Autodesk Fusion 360 part; units mm, degrees
(part 2 of 2)
sketch "Sketch11 (2)" plane through (0, 0, 48.175) normal (0, 0, 1) x (-1, 0, 0)
  line L0 (-289.1, 4) -> (-319.1, 4)
  line L1 (-319.1, 4) -> (-319.1, 214)
  line L2 (-319.1, 214) -> (-289.1, 214)
  line L3 (-289.1, 214) -> (-289.1, 4)
  line L4 (-362.3136, 6.0325) -> (-387.8522, 6.0325)
  line L5 (-387.8522, 6.0325) -> (-387.8522, 6.8243)
  line L6 (-387.8522, 6.8243) -> (-400.7794, 11.0064)
  line L7 (-400.7794, 11.0064) -> (-404.4624, 13.6097)
  line L8 (-404.4624, 13.6097) -> (-401.1196, 16.5087)
  line L9 (-401.1196, 16.5087) -> (-390.396, 19.9107)
  arc A0 (-390.396, 19.9107) -> (-390.6158, 20.6037) centre (-390.5059, 20.2572) ccw
  line L10 (-390.6158, 20.6037) -> (-390.6158, 41.3132)
  line L11 (-390.6158, 41.3132) -> (-389.869, 42.5841)
  line L12 (-389.869, 42.5841) -> (-389.869, 50.7734)
  line L13 (-389.869, 50.7734) -> (-390.2857, 50.7734)
  spline S0 degree 5 poles (-390.2857, 50.7734) (-390.2828, 50.705) (-390.2784, 50.5702) (-390.2765, 50.3743) (-390.2832, 50.1256) (-390.3073, 49.8363) (-390.3474, 49.5695) (-390.4037, 49.326) (-390.4762, 49.1069) (-390.5636, 48.9124) (-390.6642, 48.7426) (-390.7753, 48.5968) (-390.8943, 48.4742) (-391.0189, 48.374) (-391.1473, 48.2953) (-391.2783, 48.2369) (-391.3847, 48.2058) (-391.4654, 48.1911) (-391.5195, 48.185) (-391.5467, 48.1829) knots -1 -1 -1 -1 -1 -1 -0.933333 -0.866667 -0.8 -0.733333 -0.666667 -0.6 -0.533333 -0.466667 -0.4 -0.333333 -0.266667 -0.2 -0.133333 -0.066667 0 0 0 0 0 0
  line L14 (-391.5467, 48.1829) -> (-396.3987, 48.1829)
  spline S1 degree 5 poles (-396.3987, 48.1829) (-396.4412, 48.1832) (-396.5253, 48.1877) (-396.6489, 48.2065) (-396.8084, 48.2552) (-396.9988, 48.3556) (-397.1797, 48.4948) (-397.3504, 48.6711) (-397.5092, 48.8811) (-397.6541, 49.1201) (-397.7831, 49.3821) (-397.8939, 49.6613) (-397.9848, 49.952) (-398.0548, 50.2496) (-398.104, 50.551) (-398.1331, 50.8546) (-398.1438, 51.1591) (-398.1381, 51.4639) (-398.1183, 51.7675) (-398.0869, 52.0681) (-398.0463, 52.3623) (-397.9988, 52.6463) (-397.946, 52.916) (-397.8892, 53.168) (-397.8286, 53.3999) (-397.7634, 53.611) (-397.6921, 53.8022) (-397.6123, 53.9753) (-397.5222, 54.1324) (-397.4199, 54.2753) (-397.3046, 54.4051) (-397.2016, 54.4991) (-397.1182, 54.5641) (-397.06, 54.605) (-397.0302, 54.6249) knots -1 -1 -1 -1 -1 -1 -0.966667 -0.933333 -0.9 -0.866667 -0.833333 -0.8 -0.766667 -0.733333 -0.7 -0.666667 -0.633333 -0.6 -0.566667 -0.533333 -0.5 -0.466667 -0.433333 -0.4 -0.366667 -0.333333 -0.3 -0.266667 -0.233333 -0.2 -0.166667 -0.133333 -0.1 -0.066667 -0.033333 0 0 0 0 0 0
  line L15 (-397.0302, 54.6249) -> (-391.0395, 54.6249)
  spline S2 degree 5 poles (-391.0395, 54.6249) (-391.0196, 54.5925) (-390.9803, 54.5265) (-390.9226, 54.4242) (-390.8482, 54.2808) (-390.7599, 54.0891) (-390.6766, 53.8841) (-390.5987, 53.6646) (-390.5263, 53.4305) (-390.4591, 53.1824) (-390.3967, 52.9217) (-390.3502, 52.7038) (-390.3173, 52.5354) (-390.2961, 52.4211) (-390.2857, 52.3633) knots -1 -1 -1 -1 -1 -1 -0.9 -0.8 -0.7 -0.6 -0.5 -0.4 -0.3 -0.2 -0.1 0 0 0 0 0 0
  line L16 (-390.2857, 52.3633) -> (-389.9496, 52.3633)
  line L17 (-389.9496, 52.3633) -> (-389.9505, 52.7079)
  line L18 (-389.9505, 52.7079) -> (-389.9505, 61.1725)
  spline S3 degree 5 poles (-389.9505, 61.1725) (-389.9574, 61.1784) (-389.9798, 61.1969) (-390.0205, 61.2265) (-390.0836, 61.2661) (-390.1737, 61.3196) (-390.2816, 61.3926) (-390.3919, 61.4876) (-390.5004, 61.6101) (-390.6038, 61.7602) (-390.6996, 61.933) (-390.7861, 62.1204) (-390.8622, 62.3125) (-390.927, 62.4996) (-390.9803, 62.6732) (-391.0219, 62.828) (-391.0519, 62.9611) (-391.0668, 63.0492) (-391.0729, 63.1049) (-391.0747, 63.1374) (-391.075, 63.1525) knots -0.77292 -0.77292 -0.77292 -0.77292 -0.77292 -0.77292 -0.75 -0.7 -0.65 -0.6 -0.55 -0.5 -0.45 -0.4 -0.35 -0.3 -0.25 -0.2 -0.15 -0.1 -0.05 0 0 0 0 0 0
  spline S4 degree 5 poles (-391.075, 63.1525) (-391.076, 63.2134) (-391.0784, 63.3525) (-391.0827, 63.5721) (-391.0896, 63.8767) (-391.1002, 64.2749) (-391.1133, 64.7103) (-391.1281, 65.1725) (-391.1444, 65.6712) (-391.1621, 66.2157) (-391.1809, 66.8139) (-391.2007, 67.4704) (-391.2214, 68.1843) (-391.243, 68.9483) (-391.2656, 69.7464) (-391.2898, 70.5518) (-391.3158, 71.3289) (-391.344, 72.0401) (-391.3744, 72.6507) (-391.4063, 73.1351) (-391.4381, 73.482) (-391.4674, 73.701) (-391.4903, 73.827) (-391.5015, 73.9279) (-391.4957, 74.0802) (-391.4698, 74.337) (-391.4238, 74.7122) (-391.3598, 75.1937) (-391.2811, 75.7505) (-391.1914, 76.3431) (-391.0939, 76.9317) (-390.9902, 77.4855) (-390.8799, 77.9908) (-390.7613, 78.4459) (-390.6319, 78.8575) (-390.4889, 79.2371) (-390.3301, 79.5967) (-390.1543, 79.9453) (-389.9622, 80.2849) (-389.7556, 80.6117) (-389.5364, 80.9182) (-389.306, 81.1959) (-389.0641, 81.4368) (-388.8079, 81.6362) (-388.5328, 81.7926) (-388.2336, 81.9077) (-387.9064, 81.9855) (-387.5495, 82.0319) (-387.165, 82.0543) (-386.7578, 82.0608) (-386.3345, 82.0591) (-385.9022, 82.0552) (-385.4676, 82.0533) (-385.0359, 82.0538) (-384.6109, 82.0543) (-384.1971, 82.0514) (-383.8005, 82.0428) (-383.4312, 82.0288) (-383.1037, 82.0144) (-382.8401, 82.0111) (-382.6594, 82.0319) (-382.5684, 82.0854) (-382.5488, 82.169) (-382.559, 82.2687) (-382.5646, 82.3519) (-382.563, 82.4147) (-382.5593, 82.4568) (-382.5568, 82.4778) knots -0.96593682 -0.96593682 -0.96593682 -0.96593682 -0.96593682 -0.96593682 -0.95384615 -0.93846154 -0.92307692 -0.90769231 -0.89230769 -0.87692308 -0.86153846 -0.84615385 -0.83076923 -0.81538462 -0.8 -0.78461538 -0.76923077 -0.75384615 -0.73846154 -0.72307692 -0.70769231 -0.69230769 -0.67692308 -0.66153846 -0.64615385 -0.63076923 -0.61538462 -0.6 -0.58461538 -0.56923077 -0.55384615 -0.53846154 -0.52307692 -0.50769231 -0.49230769 -0.47692308 -0.46153846 -0.44615385 -0.43076923 -0.41538462 -0.4 -0.38461538 -0.36923077 -0.35384615 -0.33846154 -0.32307692 -0.30769231 -0.29230769 -0.27692308 -0.26153846 -0.24615385 -0.23076923 -0.21538462 -0.2 -0.18461538 -0.16923077 -0.15384615 -0.13846154 -0.12307692 -0.10769231 -0.09230769 -0.07692308 -0.06153846 -0.04615385 -0.03076923 -0.01538462 0 0 0 0 0 0
  line L19 (-382.5568, 82.4778) -> (-382.673, 241.7066)
  line L20 (-382.673, 241.7066) -> (-366.4147, 241.7185)
  line L21 (-366.4147, 241.7185) -> (-366.3062, 93.0229)
  spline S5 degree 5 poles (-366.3062, 93.0229) (-366.2846, 93.0312) (-366.2188, 93.0608) (-366.0959, 93.134) (-365.8932, 93.2873) (-365.5824, 93.5536) (-365.1849, 93.8948) (-364.7435, 94.2418) (-364.2682, 94.5576) (-363.7673, 94.8157) (-363.2471, 95.0039) (-362.712, 95.1199) (-362.1658, 95.1683) (-361.6114, 95.1576) (-361.0522, 95.0971) (-360.4919, 94.9934) (-359.9353, 94.848) (-359.3882, 94.6593) (-358.8567, 94.4239) (-358.3475, 94.1384) (-357.8674, 93.8004) (-357.4229, 93.4106) (-357.0208, 92.9738) (-356.6667, 92.4989) (-356.3653, 91.9969) (-356.1199, 91.4799) (-355.9313, 90.9599) (-355.798, 90.4477) (-355.7154, 89.9513) (-355.6759, 89.4755) (-355.6713, 89.0222) (-355.6936, 88.5902) (-355.7373, 88.1762) (-355.8004, 87.7738) (-355.8859, 87.3747) (-355.9991, 86.9709) (-356.1458, 86.5564) (-356.3303, 86.1297) (-356.553, 85.6961) (-356.8092, 85.2687) (-357.091, 84.8639) (-357.389, 84.4988) (-357.6939, 84.1868) (-357.9979, 83.9346) (-358.2969, 83.7381) (-358.5478, 83.6074) (-358.7368, 83.5228) (-358.8668, 83.4687) (-358.9397, 83.4393) (-358.9561, 83.4328) knots -0.950494 -0.950494 -0.950494 -0.950494 -0.950494 -0.950494 -0.94 -0.92 -0.9 -0.88 -0.86 -0.84 -0.82 -0.8 -0.78 -0.76 -0.74 -0.72 -0.7 -0.68 -0.66 -0.64 -0.62 -0.6 -0.58 -0.56 -0.54 -0.52 -0.5 -0.48 -0.46 -0.44 -0.42 -0.4 -0.38 -0.36 -0.34 -0.32 -0.3 -0.28 -0.26 -0.24 -0.22 -0.2 -0.18 -0.16 -0.14 -0.12 -0.1 -0.08 -0.074178 -0.074178 -0.074178 -0.074178 -0.074178 -0.074178
  line L22 (-358.9561, 83.4328) -> (-359.4097, 83.2583)
  spline S6 degree 5 poles (-359.4097, 83.2583) (-359.4139, 83.2568) (-359.4729, 83.2345) (-359.5862, 83.1916) (-359.6985, 83.1487) (-359.81, 83.1056) (-359.9166, 83.0639) (-359.9697, 83.043) knots -0.041525 -0.041525 -0.041525 -0.041525 -0.041525 -0.041525 -0.04 -0.02 0 0 0 0 0 0
  spline S7 degree 5 poles (-359.9697, 83.043) (-359.958, 82.9935) (-359.9278, 82.8821) (-359.8622, 82.6775) (-359.7337, 82.3297) (-359.5055, 81.771) (-359.2118, 81.0929) (-358.8574, 80.3045) (-358.4508, 79.4224) (-358.0035, 78.4687) (-357.5291, 77.4686) (-357.0428, 76.4482) (-356.5602, 75.4327) (-356.0968, 74.4439) (-355.6671, 73.4983) (-355.2837, 72.6045) (-354.9569, 71.7634) (-354.6951, 70.9706) (-354.5046, 70.219) (-354.3894, 69.5005) (-354.3516, 68.808) (-354.391, 68.1384) (-354.5054, 67.4925) (-354.6905, 66.8732) (-354.9403, 66.2847) (-355.2464, 65.7307) (-355.5989, 65.2134) (-355.9865, 64.7329) (-356.3978, 64.2876) (-356.8218, 63.8741) (-357.2495, 63.4874) (-357.674, 63.1207) (-358.0905, 62.7671) (-358.4957, 62.4196) (-358.8875, 62.0728) (-359.2647, 61.7233) (-359.5543, 61.4403) (-359.7646, 61.2258) (-359.9018, 61.0819) (-359.9697, 61.0097) knots -1 -1 -1 -1 -1 -1 -0.971429 -0.942857 -0.914286 -0.885714 -0.857143 -0.828571 -0.8 -0.771429 -0.742857 -0.714286 -0.685714 -0.657143 -0.628571 -0.6 -0.571429 -0.542857 -0.514286 -0.485714 -0.457143 -0.428571 -0.4 -0.371429 -0.342857 -0.314286 -0.285714 -0.257143 -0.228571 -0.2 -0.171429 -0.142857 -0.114286 -0.085714 -0.057143 -0.028571 0 0 0 0 0 0
  line L23 (-359.9697, 61.0097) -> (-359.9697, 35.6695)
  line L24 (-359.9697, 35.6695) -> (-332.3207, 27.7023)
  line L25 (-332.3207, 27.7023) -> (-325.7445, 21.4703)
  line L26 (-325.7445, 21.4703) -> (-326.0635, 21.1597)
  line L27 (-326.0635, 21.1597) -> (-333.1, 13.7167)
  spline S8 degree 5 poles (-333.1, 13.7167) (-333.3878, 13.6343) (-333.9657, 13.4696) (-334.8388, 13.2226) (-336.0158, 12.8932) (-337.5089, 12.4816) (-339.0245, 12.0695) (-340.5633, 11.6563) (-342.1264, 11.2407) (-343.7147, 10.8206) (-345.3286, 10.394) (-346.9663, 9.9592) (-348.6228, 9.5161) (-350.2888, 9.0666) (-351.9486, 8.6156) (-353.5804, 8.1713) (-355.1586, 7.7439) (-356.6573, 7.3442) (-358.0528, 6.9821) (-359.3264, 6.6655) (-360.4685, 6.3988) (-361.274, 6.2265) (-361.8173, 6.1205) (-362.1526, 6.0601) (-362.3136, 6.0325) knots -1 -1 -1 -1 -1 -1 -0.95 -0.9 -0.85 -0.8 -0.75 -0.7 -0.65 -0.6 -0.55 -0.5 -0.45 -0.4 -0.35 -0.3 -0.25 -0.2 -0.15 -0.1 -0.05 0 0 0 0 0 0
  line L28 (-285.1, 297.942) -> (-407.924, 297.942)
  line L29 (-407.924, 297.942) -> (-407.924, 0)
  line L30 (-407.924, 0) -> (-285.1, 0)
  line L31 (-285.1, 0) -> (-285.1, 297.942)
  line L32 (-385.1102, 253.2) -> (-385.1102, 92)
  line L33 (-385.1102, 92) -> (-404.9102, 92)
  line L34 (-404.9102, 92) -> (-404.9102, 253.2)
  line L35 (-404.9102, 253.2) -> (-385.1102, 253.2)
  line L36 (-324.1, 37.2288) -> (-340.1, 37.2288)
  line L37 (-340.1, 37.2288) -> (-340.1, 250.1308)
  line L38 (-340.1, 250.1308) -> (-324.1, 250.1308)
  line L39 (-324.1, 250.1308) -> (-324.1, 37.2288)
  dimension "d255" = 16
  dimension "d256" = 212.902
  dimension "d257" = 5
  dimension "d258" = 7
  constraint horizontal L36
  constraint vertical L37
  constraint horizontal L38
  constraint vertical L39
  measures "d255" distance of L36.start L36.end
  measures "d256" distance of L36.start L38.end
  measures "d257" distance of L1 L39
  measures "d258" distance of L24 L36.end
extrude "Extrude14" [suppressed]
sketch "Sketch12" plane through (0, 0, 3.175) normal (0, 0, 1) x (-1, 0, 0)
  line L0 (0, 0) -> (0, 297.942)
  line L1 (0, 297.942) -> (-407.924, 297.942)
  line L2 (-407.924, 297.942) -> (-407.924, 0)
  line L3 (-407.924, 0) -> (0, 0)
  line L4 (-289.1, 4) -> (-319.1, 4)
  line L5 (-289.1, 214) -> (-289.1, 4)
  line L6 (-319.1, 4) -> (-319.1, 214)
  line L7 (-319.1, 214) -> (-289.1, 214)
extrude "Extrude15" [suppressed]
split "Split1" [suppressed]
copy_body "Body->Comp1" [suppressed] in component "Upper-Caliper-Holder"
copy_body "Body->Comp2" [suppressed] in component "Lower-Caliper-Holder"
equation "d240 = -ComponentWallWidth"
equation "d256 = 8.38 in + SmallTolerence"
equation "ComponentWallWidth = 4 mm"
equation "SmallTolerence = 0.05 mm"
